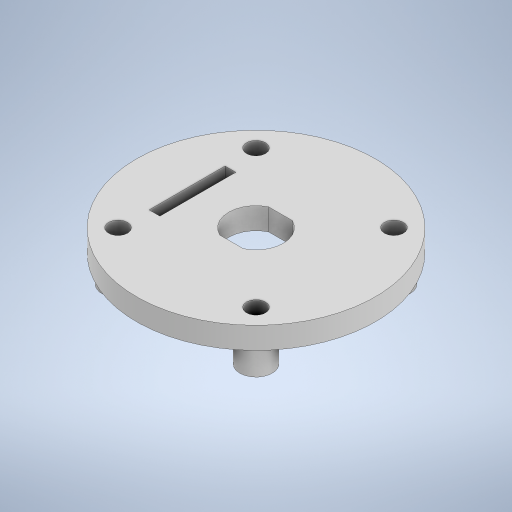
# Autodesk Inventor part: bevestigingpot
Saved by Autodesk Inventor 2024 (Build 280153000, 153)
## iProperties
Created: 2023-11-06
Part Number: bevestigingpot
Material: Generic
Document SubType Name: Modeling
Designer: Nikita
Density: 1 g/cm^3
Appearance: Default
Author: Nikita
Autodesk Inventor part; units mm, degrees
ref_plane "YZ Plane" through (0, 0, 0) normal (1, 0, 0) x (0, 1, 0)
ref_plane "XZ Plane" through (0, 0, 0) normal (0, 1, 0) x (-1, 0, 0)
ref_plane "XY Plane" through (0, 0, 0) normal (0, 0, 1) x (1, 0, 0)
sketch "Sketch1" plane through (0, 0, 0) normal (0, 1, 0) x (-1, 0, 0)
  circle A0 centre (0, 0) radius 22
  dimension "d0" = 44
  constraints: 1 centre point, 1 coincident
  measures "d0" diameter of A0
extrude "Extrusion1" add sketch "Sketch1" along normal blind 4
sketch "Sketch2" plane through (0, 4, 0) normal (0, 1, 0) x (1, 0, 0)
  line L0 (0, 0) -> (-12.7, 0) construction
  line L1 (0, 0) -> (12.7, 0) construction
  line L2 (-12.7, 0) -> (-12.7, 12.7) construction
  line L3 (-12.7, 12.7) -> (12.7, 12.7) construction
  circle A0 centre (-12.7, 12.7) radius 1.75
  dimension "d3" = 12.7
  dimension "d4" = 12.7
  dimension "d5" = 12.7
  dimension "d6" = 3.5
  constraints: 8 end point, 2 horizontal, 1 centre point, 1 coincident, 1 perpendicular, 1 vertical
  measures "d3" distance of L0.start L0.end
  measures "d4" distance of L0.start L1.end
  measures "d5" distance of L0.end L2.end
  measures "d6" diameter of A0
extrude "Extrusion2" cut sketch "Sketch2" against normal blind 4
pattern_circular "Circular Pattern1" count 4 over 360 about axis through (0, 0, 0) along (0, 1, 0) of "Extrusion2"
sketch "Sketch3" plane through (0, 4, 0) normal (0, 1, 0) x (1, 0, 0)
  line L0 (0, 0) -> (-12.7, 0) construction
  line L1 (-12.7, 0) -> (-12.7, 7) construction
  line L2 (-12.7, 7) -> (-10.7, 7) construction
  line L3 (-10.7, 7) -> (-10.7, -7) construction
  line L4 (-10.7, -7) -> (-12.7, -7)
  line L5 (-12.7, -7) -> (-12.7, 7)
  line L6 (-12.7, 7) -> (-10.7, 7)
  line L7 (-10.7, 7) -> (-10.7, -7)
  dimension "d12" = 12.7
  dimension "d13" = 7
  dimension "d14" = 2
  dimension "d15" = 14
  constraints: 16 end point, 4 perpendicular, 2 horizontal, 2 parallel
  measures "d12" distance of L0.start L0.end
  measures "d13" distance of L0.end L1.end
  measures "d14" distance of L1.end L2.end
  measures "d15" distance of L2.end L3.end
extrude "Extrusion3" cut sketch "Sketch3" against normal blind 4
sketch "Sketch4" plane through (0, 4, 0) normal (0, 1, 0) x (1, 0, 0)
  circle A0 centre (-12.7, 12.7) radius 1.75 projected
  line L0 (0, 0) -> (-12.7, 12.7)
  line L1 (-4.5, 0) -> (-4.5, -2.1794) construction
  line L2 (0, 4.5) -> (0, -4.5) construction
  line L3 (-2.1794, 4.5) -> (2.1794, 4.5)
  line L4 (-2.1794, -4.5) -> (2.1794, -4.5)
  arc A1 (2.1794, -4.5) -> (2.1794, 4.5) centre (0, 0) ccw
  arc A2 (-2.1794, 4.5) -> (-2.1794, -4.5) centre (0, 0) ccw
  dimension "d21" = 4.5
  dimension "d22" = 9
  constraints: 10 end point, 5 point on circle, 2 centre point, 1 coincident, 1 horizontal, 1 parallel
  measures "d21" distance of L0.start L2.start
  measures "d22" distance of L2.start L2.end
extrude "Extrusion4" cut sketch "Sketch4" against normal blind 4 contours L3 A1 L4 A2
sketch "Sketch5" plane through (0, 0, 0) normal (0, -1, 0) x (1, 0, 0)
  circle A0 centre (-12.7, 12.7) radius 1.75 projected
  circle A1 centre (-12.7, 12.7) radius 3
  circle A2 centre (-12.7, 12.7) radius 1.75
  point P0 (0, 0)
  dimension "d25" = 6
  constraints: 2 centre point, 2 coincident, 1 concentric
  measures "d25" diameter of A1
extrude "Extrusion5" add sketch "Sketch5" along normal blind 5
pattern_circular "Circular Pattern2" count 4 over 360 about axis through (0, 0, 0) along (0, 1, 0) of "Extrusion5"
body "Solid1"
